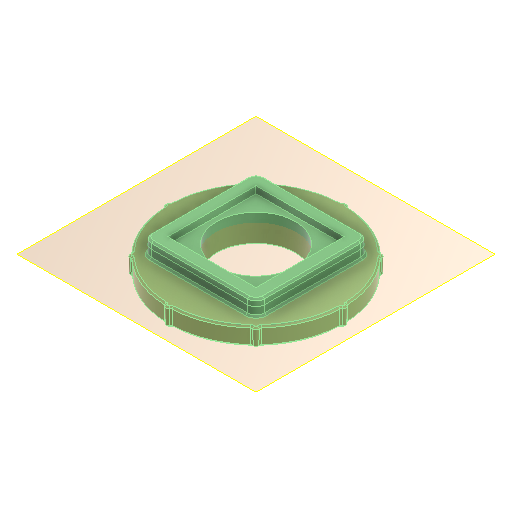
# Autodesk Inventor part: 20_Cube_4_insert_beamsplitter_20mm
Saved by Autodesk Inventor 2025.1 (Build 291241000, 241)
## iProperties
Created: 2024-10-03
Part Number: 20_Cube_4_insert_beamsplitter_20mm
Material: Generic
Document SubType Name: Modeling
Designer: diederichbenedict
Density: 1 g/cm^3
Appearance: Smooth - Dark Forest Green
Author: diederichbenedict
Autodesk Inventor part; units mm, degrees
ref_plane "YZ Plane" through (0, 0, 0) normal (1, 0, 0) x (0, 1, 0)
ref_plane "Work Plane1" through (0, 0, 0) normal (0, 0, 1) x (1, 0, 0)
sketch "Sketch1" plane through (0, 0, 0) normal (0, 0, 1) x (1, 0, 0)
  arc A0 (1.5114, -4.263) -> (1.1737, -4.342) centre (1.4126, -4.6023) ccw projected
  arc A1 (-11.5885, -9.6282) -> (1.1737, -4.342) centre (-12.45, 10.5) ccw projected
  arc A2 (-11.5885, -9.6282) -> (-11.8831, -9.8112) centre (-11.5734, -9.9813) ccw projected
  arc A3 (-13.0169, -9.8112) -> (-11.8831, -9.8112) centre (-12.45, -9.5) ccw projected
  arc A4 (-13.0169, -9.8112) -> (-13.3115, -9.6282) centre (-13.3266, -9.9813) ccw projected
  arc A5 (-26.0737, -4.342) -> (-13.3115, -9.6282) centre (-12.45, 10.5) ccw projected
  arc A6 (-26.0737, -4.342) -> (-26.4114, -4.263) centre (-26.3126, -4.6023) ccw projected
  arc A7 (-27.213, -3.4614) -> (-26.4114, -4.263) centre (-26.5921, -3.6421) ccw projected
  arc A8 (-27.213, -3.4614) -> (-27.292, -3.1237) centre (-27.5523, -3.3626) ccw projected
  arc A9 (-32.5782, 9.6385) -> (-27.292, -3.1237) centre (-12.45, 10.5) ccw projected
  arc A10 (-32.5782, 9.6385) -> (-32.7612, 9.9331) centre (-32.9312, 9.6234) ccw projected
  arc A11 (-32.7612, 11.0669) -> (-32.7612, 9.9331) centre (-32.45, 10.5) ccw projected
  arc A12 (-32.7612, 11.0669) -> (-32.5782, 11.3615) centre (-32.9312, 11.3766) ccw projected
  arc A13 (-27.292, 24.1237) -> (-32.5782, 11.3615) centre (-12.45, 10.5) ccw projected
  arc A14 (-27.292, 24.1237) -> (-27.213, 24.4614) centre (-27.5523, 24.3626) ccw projected
  arc A15 (-26.4114, 25.263) -> (-27.213, 24.4614) centre (-26.5921, 24.6421) ccw projected
  arc A16 (-26.4114, 25.263) -> (-26.0737, 25.342) centre (-26.3126, 25.6023) ccw projected
  arc A17 (-13.3115, 30.6282) -> (-26.0737, 25.342) centre (-12.45, 10.5) ccw projected
  arc A18 (-13.3115, 30.6282) -> (-13.0169, 30.8112) centre (-13.3266, 30.9812) ccw projected
  arc A19 (-11.8831, 30.8112) -> (-13.0169, 30.8112) centre (-12.45, 30.5) ccw projected
  arc A20 (-11.8831, 30.8112) -> (-11.5885, 30.6282) centre (-11.5734, 30.9812) ccw projected
  arc A21 (1.1737, 25.342) -> (-11.5885, 30.6282) centre (-12.45, 10.5) ccw projected
  arc A22 (1.1737, 25.342) -> (1.5114, 25.263) centre (1.4126, 25.6023) ccw projected
  arc A23 (2.313, 24.4614) -> (1.5114, 25.263) centre (1.6921, 24.6421) ccw projected
  arc A24 (2.313, 24.4614) -> (2.392, 24.1237) centre (2.6523, 24.3626) ccw projected
  arc A25 (7.6782, 11.3615) -> (2.392, 24.1237) centre (-12.45, 10.5) ccw projected
  arc A26 (7.6782, 11.3615) -> (7.8612, 11.0669) centre (8.0313, 11.3766) ccw projected
  arc A27 (7.8612, 9.9331) -> (7.8612, 11.0669) centre (7.55, 10.5) ccw projected
  arc A28 (7.8612, 9.9331) -> (7.6782, 9.6385) centre (8.0313, 9.6234) ccw projected
  arc A29 (2.392, -3.1237) -> (7.6782, 9.6385) centre (-12.45, 10.5) ccw projected
  arc A30 (2.392, -3.1237) -> (2.313, -3.4614) centre (2.6523, -3.3626) ccw projected
  arc A31 (1.5114, -4.263) -> (2.313, -3.4614) centre (1.6921, -3.6421) ccw projected
  arc A32 (-36.6117, 25.3443) -> (-37.35, 24.9048) centre (-36.85, 24.9048) ccw projected
  line L0 (-37.35, 24.9048) -> (-37.35, -3.9048) projected
  arc A33 (-37.35, -3.9048) -> (-36.6117, -4.3443) centre (-36.85, -3.9048) ccw projected
  line L1 (-36.6117, -4.3443) -> (-34.9957, -3.4684) projected
  arc A34 (-34.9957, -4.4161) -> (-34.9957, -3.4684) centre (-34.4238, -3.9422) ccw projected
  line L2 (-34.9957, -4.4161) -> (-37.35, -5.6921) projected
  line L3 (-37.35, -5.6921) -> (-37.35, -6.7071) projected
  arc A35 (-37.35, -6.7071) -> (-36.4964, -7.0607) centre (-36.85, -6.7071) ccw projected
  line L4 (-36.4964, -7.0607) -> (-35.9358, -6.5) projected
  line L5 (-35.9358, -6.5) -> (-33.45, -6.5) projected
  line L6 (-33.45, -6.5) -> (-29.45, -10.5) projected
  line L7 (-29.45, -10.5) -> (-29.3819, -14.4) projected
  line L8 (4.4819, -14.4) -> (-29.3819, -14.4) projected
  line L9 (4.4819, -14.4) -> (4.55, -10.5) projected
  line L10 (8.55, -6.5) -> (4.55, -10.5) projected
  line L11 (11.0358, -6.5) -> (8.55, -6.5) projected
  line L12 (11.5964, -7.0607) -> (11.0358, -6.5) projected
  arc A36 (11.5964, -7.0607) -> (12.45, -6.7071) centre (11.95, -6.7071) ccw projected
  line L13 (12.45, -5.6921) -> (12.45, -6.7071) projected
  line L14 (12.45, -5.6921) -> (10.0957, -4.4161) projected
  arc A37 (10.0957, -3.4684) -> (10.0957, -4.4161) centre (9.5238, -3.9422) ccw projected
  line L15 (10.0957, -3.4684) -> (11.7117, -4.3443) projected
  arc A38 (11.7117, -4.3443) -> (12.45, -3.9048) centre (11.95, -3.9048) ccw projected
  line L16 (12.45, -3.9048) -> (12.45, 24.9048) projected
  arc A39 (12.45, 24.9048) -> (11.7117, 25.3443) centre (11.95, 24.9048) ccw projected
  line L17 (11.7117, 25.3443) -> (10.0957, 24.4684) projected
  arc A40 (10.0957, 25.4161) -> (10.0957, 24.4684) centre (9.5238, 24.9422) ccw projected
  line L18 (10.0957, 25.4161) -> (12.45, 26.6921) projected
  line L19 (12.45, 26.6921) -> (12.45, 27.7071) projected
  arc A41 (12.45, 27.7071) -> (11.5964, 28.0607) centre (11.95, 27.7071) ccw projected
  line L20 (11.5964, 28.0607) -> (11.0358, 27.5) projected
  line L21 (11.0358, 27.5) -> (8.55, 27.5) projected
  line L22 (8.55, 27.5) -> (4.55, 31.5) projected
  line L23 (4.55, 31.5) -> (4.4819, 35.4) projected
  line L24 (-29.3819, 35.4) -> (4.4819, 35.4) projected
  line L25 (-29.3819, 35.4) -> (-29.45, 31.5) projected
  line L26 (-33.45, 27.5) -> (-29.45, 31.5) projected
  line L27 (-35.9358, 27.5) -> (-33.45, 27.5) projected
  line L28 (-36.4964, 28.0607) -> (-35.9358, 27.5) projected
  arc A42 (-36.4964, 28.0607) -> (-37.35, 27.7071) centre (-36.85, 27.7071) ccw projected
  line L29 (-37.35, 27.7071) -> (-37.35, 26.6921) projected
  line L30 (-37.35, 26.6921) -> (-34.9957, 25.4161) projected
  arc A43 (-34.9957, 24.4684) -> (-34.9957, 25.4161) centre (-34.4238, 24.9422) ccw projected
  line L31 (-34.9957, 24.4684) -> (-36.6117, 25.3443) projected
  circle A44 centre (4.05, 27) radius 1.4 projected
  circle A45 centre (4.05, -6) radius 1.4 projected
  circle A46 centre (-28.95, 27) radius 1.4 projected
  circle A47 centre (-28.95, -6) radius 1.4 projected
  point P0 (0, 0)
ref_plane "Work Plane2" through (-32.95, -10, -4.2) normal (0, 0, 1) x (1, 0, 0)
extrude "Extrusion1" add sketch "Sketch1" against normal up to surface (4.2 mm away) draft -2 contours A0 A1 A2 A3 A4 A5 A6 A7 A8 A9 A10 A11 A12 A13 A14 A15 A16 A17 A18 A19 A20 A21 A22 A23 A24 A25 A26 A27 A28 A29 A30 A31
sketch "Sketch2" plane through (0, 0, 0) normal (0, 0, 1) x (1, 0, 0)
  line L0 (-2.45, 0.5) -> (-22.45, 0.5) projected
  line L1 (-2.45, 0.5) -> (-2.45, 20.5) projected
  line L2 (-22.45, 20.5) -> (-2.45, 20.5) projected
  line L3 (-22.45, 0.5) -> (-22.45, 20.5) projected
  line L4 (0.55, 21.5) -> (0.55, -0.5)
  line L5 (-1.45, -2.5) -> (-23.45, -2.5)
  line L6 (-25.45, -0.5) -> (-25.45, 21.5)
  line L7 (-23.45, 23.5) -> (-1.45, 23.5)
  arc A0 (0.55, 21.5) -> (-1.45, 23.5) centre (-1.45, 21.5) ccw
  arc A1 (-23.45, 23.5) -> (-25.45, 21.5) centre (-23.45, 21.5) ccw
  arc A2 (-25.45, -0.5) -> (-23.45, -2.5) centre (-23.45, -0.5) ccw
  arc A3 (-1.45, -2.5) -> (0.55, -0.5) centre (-1.45, -0.5) ccw
  point P0 (0, 0)
  dimension "d2" = 3
  dimension "d3" = 2
  constraints: 8 end point, 8 point on circle, 8 tangent, 4 centre point, 3 equal radius, 3 other
  measures "d2" distance between parallel lines of L1 L4
  measures "d3" radius of A0
ref_plane "Work Plane3" through (-22.45, 0.5, 2) normal (0, 0, -1) x (0, 1, 0)
extrude "Extrusion2" add sketch "Sketch2" along normal up to surface (2 mm away) contours L0 L3 L2 L1 | L4 A3 L5 A2 L6 A1 L7 A0
sketch "Sketch3" plane through (-23.45, -2.5, 2) normal (0, 0, 1) x (1, 0, 0)
  line L0 (21, 3) -> (1, 3) projected
  line L1 (21, 3) -> (21, 23) projected
  line L2 (1, 23) -> (21, 23) projected
  line L3 (1, 3) -> (1, 23) projected
  arc A0 (0, 26) -> (-2, 24) centre (0, 24) ccw projected
  line L4 (-2, 24) -> (-2, 2) projected
  arc A1 (-2, 2) -> (0, 0) centre (0, 2) ccw projected
  line L5 (0, 0) -> (22, 0) projected
  arc A2 (22, 0) -> (24, 2) centre (22, 2) ccw projected
  line L6 (24, 2) -> (24, 24) projected
  arc A3 (24, 24) -> (22, 26) centre (22, 24) ccw projected
  line L7 (22, 26) -> (0, 26) projected
  point P0 (23.45, 2.5)
extrude "Extrusion3" add sketch "Sketch3" along normal blind 1.5 draft -4
chamfer "Chamfer1" distance 0.4 angle 45 80 edges at (-20.1037, 28.9776, -4.2) (-13.0628, 30.5565, -4.2) (-12.45, 31, -4.2) (-11.8372, 30.5565, -4.2) (-4.7963, 28.9776, -4.2) (1.2988, 25.1154, -4.2) (2.0457, 24.9957, -4.2) (2.1654, 24.2488, -4.2) (6.0276, 18.1537, -4.2) (7.6065, 11.1128, -4.2) (8.05, 10.5, -4.2) (7.6065, 9.8872, -4.2) (6.0276, 2.8463, -4.2) (2.1654, -3.2488, -4.2) (2.0457, -3.9957, -4.2) (1.2988, -4.1154, -4.2) (-4.7963, -7.9776, -4.2) (-11.8372, -9.5565, -4.2) (-12.45, -10, -4.2) (-13.0628, -9.5565, -4.2) (-20.1037, -7.9776, -4.2) (-26.1988, -4.1154, -4.2) (-26.9457, -3.9957, -4.2) (-27.0654, -3.2488, -4.2) (-30.9276, 2.8463, -4.2) (-32.5065, 9.8872, -4.2) (-32.95, 10.5, -4.2) (-32.5065, 11.1128, -4.2) (-30.9276, 18.1537, -4.2) (-27.0654, 24.2488, -4.2) (-26.9457, 24.9957, -4.2) (-26.1988, 25.1154, -4.2) (-4.7402, 29.1131, 0) (-11.7598, 30.6811, 0) (-12.45, 31.1467, 0) (-13.1402, 30.6811, 0) (-20.1598, 29.1131, 0) (-26.2322, 25.2582, 0) (-27.0494, 25.0994, 0) (-27.2082, 24.2822, 0) (-31.0631, 18.2098, 0) (-32.6311, 11.1902, 0) (-33.0967, 10.5, 0) (-32.6311, 9.8098, 0) (-31.0631, 2.7902, 0) (-27.2082, -3.2822, 0) (-27.0494, -4.0994, 0) (-26.2322, -4.2582, 0) (-20.1598, -8.1131, 0) (-13.1402, -9.6811, 0) (-12.45, -10.1467, 0) (-11.7598, -9.6811, 0) (-4.7402, -8.1131, 0) (1.3322, -4.2582, 0) (2.1494, -4.0994, 0) (2.3082, -3.2822, 0) (6.1631, 2.7902, 0) (7.7311, 9.8098, 0) (8.1967, 10.5, 0) (7.7311, 11.1902, 0) (6.1631, 18.2098, 0) (2.3082, 24.2822, 0) (2.1494, 25.0994, 0) (1.3322, 25.2582, 0) (0.55, 10.5, 0) (-0.0358, -1.9142, 0) (-12.45, -2.5, 0) (-24.8642, -1.9142, 0) (-25.45, 10.5, 0) (-24.8642, 22.9142, 0) (-12.45, 23.5, 0) (-0.0358, 22.9142, 0) (-0.11, 22.84, 3.5) (0.4451, 10.5, 3.5) (-0.11, -1.84, 3.5) (-12.45, -2.3951, 3.5) (-24.79, -1.84, 3.5) (-25.3451, 10.5, 3.5) (-24.79, 22.84, 3.5) (-12.45, 23.3951, 3.5)
sketch "Sketch4" plane through (0, 0, 0) normal (0, 0, 1) x (1, 0, 0)
  arc A0 (-13.2881, 30.0821) -> (-25.704, 24.9392) centre (-12.45, 10.5) ccw projected
  arc A1 (-13.2881, 30.0821) -> (-12.5377, 30.5481) centre (-13.3266, 30.9812) ccw projected
  arc A2 (-12.3623, 30.5481) -> (-12.5377, 30.5481) centre (-12.45, 30.5) ccw projected
  arc A3 (-12.3623, 30.5481) -> (-11.6119, 30.0821) centre (-11.5734, 30.9812) ccw projected
  arc A4 (0.804, 24.9392) -> (-11.6119, 30.0821) centre (-12.45, 10.5) ccw projected
  arc A5 (0.804, 24.9392) -> (1.6642, 24.7381) centre (1.4126, 25.6023) ccw projected
  arc A6 (1.7881, 24.6142) -> (1.6642, 24.7381) centre (1.6921, 24.6421) ccw projected
  arc A7 (1.7881, 24.6142) -> (1.9892, 23.754) centre (2.6523, 24.3626) ccw projected
  arc A8 (7.1321, 11.3381) -> (1.9892, 23.754) centre (-12.45, 10.5) ccw projected
  arc A9 (7.1321, 11.3381) -> (7.5981, 10.5877) centre (8.0313, 11.3766) ccw projected
  arc A10 (7.5981, 10.4123) -> (7.5981, 10.5877) centre (7.55, 10.5) ccw projected
  arc A11 (7.5981, 10.4123) -> (7.1321, 9.6619) centre (8.0313, 9.6234) ccw projected
  arc A12 (1.9892, -2.754) -> (7.1321, 9.6619) centre (-12.45, 10.5) ccw projected
  arc A13 (1.9892, -2.754) -> (1.7881, -3.6142) centre (2.6523, -3.3626) ccw projected
  arc A14 (1.6642, -3.7381) -> (1.7881, -3.6142) centre (1.6921, -3.6421) ccw projected
  arc A15 (1.6642, -3.7381) -> (0.804, -3.9392) centre (1.4126, -4.6023) ccw projected
  arc A16 (-11.6119, -9.0821) -> (0.804, -3.9392) centre (-12.45, 10.5) ccw projected
  arc A17 (-11.6119, -9.0821) -> (-12.3623, -9.5481) centre (-11.5734, -9.9813) ccw projected
  arc A18 (-12.5377, -9.5481) -> (-12.3623, -9.5481) centre (-12.45, -9.5) ccw projected
  arc A19 (-12.5377, -9.5481) -> (-13.2881, -9.0821) centre (-13.3266, -9.9813) ccw projected
  arc A20 (-25.704, -3.9392) -> (-13.2881, -9.0821) centre (-12.45, 10.5) ccw projected
  arc A21 (-25.704, -3.9392) -> (-26.5642, -3.7381) centre (-26.3126, -4.6023) ccw projected
  arc A22 (-26.6881, -3.6142) -> (-26.5642, -3.7381) centre (-26.5921, -3.6421) ccw projected
  arc A23 (-26.6881, -3.6142) -> (-26.8892, -2.754) centre (-27.5523, -3.3626) ccw projected
  arc A24 (-32.0321, 9.6619) -> (-26.8892, -2.754) centre (-12.45, 10.5) ccw projected
  arc A25 (-32.0321, 9.6619) -> (-32.4981, 10.4123) centre (-32.9312, 9.6234) ccw projected
  arc A26 (-32.4981, 10.5877) -> (-32.4981, 10.4123) centre (-32.45, 10.5) ccw projected
  arc A27 (-32.4981, 10.5877) -> (-32.0321, 11.3381) centre (-32.9312, 11.3766) ccw projected
  arc A28 (-26.8892, 23.754) -> (-32.0321, 11.3381) centre (-12.45, 10.5) ccw projected
  arc A29 (-26.8892, 23.754) -> (-26.6881, 24.6142) centre (-27.5523, 24.3626) ccw projected
  arc A30 (-26.5642, 24.7381) -> (-26.6881, 24.6142) centre (-26.5921, 24.6421) ccw projected
  arc A31 (-26.5642, 24.7381) -> (-25.704, 24.9392) centre (-26.3126, 25.6023) ccw projected
  circle A32 centre (-12.45, 10.5) radius 19 projected
  circle A33 centre (-12.45, 10.5) radius 9
  point P0 (0, 0)
  dimension "d11" = 18
  constraints: 1 centre point, 1 coincident
  measures "d11" diameter of A33
extrude "Extrusion4" cut sketch "Sketch4" along normal through all both and the other way through all contours A33
body "Solid1"
